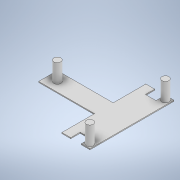
# Autodesk Inventor part: bottenplatta
Saved by Autodesk Inventor 2020 (Build 240168000, 168)
## iProperties
Created: 2020-03-24
Part Number: bottenplatta
Material: Generic
Document SubType Name: Modeling
Designer: magnu
Density: 1 g/cm^3
Appearance: Default
Mass: 50.6809 g
Surface Area: 367.3 cm^2
Volume: 50.6809 cm^3
Author: magnu
Autodesk Inventor part; units mm, degrees
ref_plane "YZ Plane" through (0, 0, 0) normal (1, 0, 0) x (0, 1, 0)
ref_plane "XZ Plane" through (0, 0, 0) normal (0, 1, 0) x (-1, 0, 0)
ref_plane "XY Plane" through (0, 0, 0) normal (0, 0, 1) x (1, 0, 0)
sketch "Sketch1" plane through (0, 0, 0) normal (0, 1, 0) x (-1, 0, 0)
  line L0 (0, 90) -> (0, -90)
  line L1 (0, -90) -> (18.6089, -90)
  line L2 (18.6089, -90) -> (18.6089, -70)
  line L3 (18.6089, -70) -> (41.1664, -70)
  line L4 (41.1664, -70) -> (41.1664, -90)
  line L5 (41.1664, -90) -> (60.3061, -90)
  line L6 (60.3061, -90) -> (60.3061, -20)
  line L7 (60.3061, -20) -> (180, -20)
  line L8 (180, -20) -> (180, 20)
  line L9 (41.1664, 70) -> (18.6089, 70)
  line L10 (18.6089, 70) -> (18.6089, 90)
  line L11 (18.6089, 90) -> (0, 90)
  line L12 (180, 20) -> (60.2637, 20)
  line L13 (60.2637, 20) -> (60.2637, 90)
  line L14 (41.1664, 70) -> (41.1664, 90)
  line L15 (41.1664, 90) -> (60.2637, 90)
  point P0 (0, 0)
  dimension "d0" = 180
  dimension "d1" = 180
  dimension "d3" = 20
  dimension "d4" = 20
  dimension "d5" = 20
  dimension "d6" = 20
  dimension "d7" = 40
  dimension "d8" = 70
  dimension "d9" = 70
  dimension "d10" = 90
  constraints: 32 end point, 10 perpendicular, 2 horizontal, 2 vertical
  measures "d0" distance of L0.start L0.end
  measures "d1" distance between parallel lines of L8 L0
  measures "d3" distance of L9.end L10.end
  measures "d4" distance of L1.end L2.end
  measures "d5" distance of L3.end L4.end
  measures "d6" distance of L9.start L14.end
  measures "d7" distance of L7.end L8.end
  measures "d8" distance of L5.end L6.end
  measures "d9" distance of L12.end L13.end
  measures "d10" distance from line of point (0, 0) L1
extrude "Extrusion1" add sketch "Sketch1" along normal blind 2
sketch "Sketch2" plane through (0, 2, 0) normal (0, 1, 0) x (1, 0, 0)
  circle A0 centre (-160, 0) radius 7.5
  circle A1 centre (-9.3045, -81) radius 7.5
  circle A2 centre (-9.3045, 81) radius 7.5
  line L0 (0, 90) -> (-18.6089, 90) projected
  line L1 (0, -90) -> (0, 90) projected
  line L2 (-18.6089, -90) -> (0, -90) projected
  line L3 (-180, 20) -> (-180, -20) projected
  point P0 (0, 0)
  dimension "d13" = 15
  dimension "d14" = 15
  dimension "d15" = 15
  dimension "d16" = 9
  dimension "d17" = 9.3045
  dimension "d18" = 9
  dimension "d19" = 9.3045
  dimension "d20" = 20
  constraints: 3 centre point
  measures "d13" diameter of A0
  measures "d14" diameter of A2
  measures "d15" diameter of A1
  measures "d16" distance from line of L0 A2.centre
  measures "d17" distance from line of L1 A2.centre
  measures "d18" distance from line of L2 A1.centre
  measures "d19" distance from line of L1 A1.centre
  measures "d20" distance from line of L3 A0.centre
extrude "Extrusion2" add sketch "Sketch2" along normal blind 40
equation "\"d4\" = d3"
equation "\"d5\" = d4"
equation "\"d6\" = d3"
equation "\"d9\" = d8"
equation "\"d14\" = d13"
equation "\"d15\" = d13"
equation "\"d18\" = d16"
equation "\"d19\" = d17"
body "Solid1"
